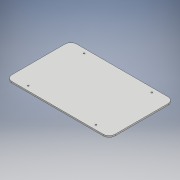
# Autodesk Inventor part: TopBoard
Saved by Autodesk Inventor 2017 (Build 210142000, 142)
## iProperties
Part Number: TopBoard
Material: 一般
Document SubType Name: Modeling
Designer: 0125r
Density: 1 g/cm^3
Appearance: 既定
Author: 0125r
Autodesk Inventor part; units mm, degrees
ref_plane "YZ Plane" through (0, 0, 0) normal (1, 0, 0) x (0, 1, 0)
ref_plane "XZ Plane" through (0, 0, 0) normal (0, 1, 0) x (-1, 0, 0)
ref_plane "XY Plane" through (0, 0, 0) normal (0, 0, 1) x (1, 0, 0)
sketch "スケッチ1" plane through (0, 0, 0) normal (0, 0, 1) x (1, 0, 0)
  line L0 (-155, -110) -> (155, -110)
  line L1 (175, -90) -> (175, 90)
  line L2 (155, 110) -> (-155, 110)
  line L3 (-175, 90) -> (-175, -90)
  line L4 (-175, -110) -> (175, 110) construction
  line L5 (175, -110) -> (-175, 110) construction
  arc A0 (175, 90) -> (155, 110) centre (155, 90) ccw
  arc A1 (155, -110) -> (175, -90) centre (155, -90) ccw
  arc A2 (-175, -90) -> (-155, -110) centre (-155, -90) ccw
  arc A3 (-155, 110) -> (-175, 90) centre (-155, 90) ccw
  circle A4 centre (115, -95) radius 2.5
  circle A5 centre (-115, -95) radius 2.5
  circle A6 centre (115, 95) radius 2.5
  circle A7 centre (-115, 95) radius 2.5
  point P0 (0, 0)
  dimension "d0" = 350
  dimension "d1" = 220
  dimension "d2" = 20
  dimension "d3" = 20
  dimension "d4" = 20
  dimension "d5" = 20
  dimension "d6" = 5
  dimension "d7" = 15
  dimension "d8" = 60
  dimension "d9" = 15
  dimension "d10" = 60
  dimension "d11" = 15
  dimension "d12" = 60
  dimension "d13" = 15
  dimension "d14" = 60
  constraints: 12 end point, 8 centre point, 8 point on circle, 8 point on line, 8 tangent, 2 midpoint, 2 parallel, 1 horizontal, 1 perpendicular
  measures "d0" distance of L4.end L5.end
  measures "d1" distance of L5.start L4.end
  measures "d2" radius of A0
  measures "d3" radius of A1
  measures "d4" radius of A2
  measures "d5" radius of A3
  measures "d6" diameter of A4
  measures "d7" distance from line of A4.centre L0
  measures "d8" distance from line of L1 A4.centre
  measures "d9" distance from line of A5.centre L0
  measures "d10" distance from line of L3 A5.centre
  measures "d11" distance from line of L2 A7.centre
  measures "d12" distance from line of L3 A7.centre
  measures "d13" distance from line of L2 A6.centre
  measures "d14" distance from line of L1 A6.centre
sketch "スケッチ2" plane through (0, 0, 0) normal (0, 0, 1) x (1, 0, 0)
  point P0 (0, 0)
sketch "スケッチ3" plane through (0, 0, 0) normal (0, 0, 1) x (1, 0, 0)
  point P0 (0, 0)
extrude "押し出し1" add sketch "スケッチ1" along normal blind 5
